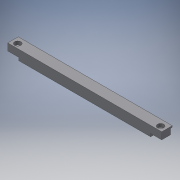
# Autodesk Inventor part: Case_bottom_front
Saved by Autodesk Inventor 2016 SP2 (Build 200236200, 236)
## iProperties
Created: 2018-06-26
Part Number: Case_bottom_front
Material: Generisch
Document SubType Name: Modeling
Designer: Nils
Density: 1 g/cm^3
Appearance: Vorgabe
Author: Nils
Autodesk Inventor part; units mm, degrees
ref_plane "YZ Plane" through (0, 0, 0) normal (1, 0, 0) x (0, 1, 0)
ref_plane "XZ Plane" through (0, 0, 0) normal (0, 1, 0) x (-1, 0, 0)
ref_plane "XY Plane" through (0, 0, 0) normal (0, 0, 1) x (1, 0, 0)
sketch "Skizze2" plane through (0, 0, 0) normal (1, 0, 0) x (0, 1, 0)
  line L0 (-333.777, 348.0872) -> (-334.0423, 350.6737)
  line L1 (-333.777, 348.0872) -> (-333.134, 341.8201)
  line L2 (-333.134, 341.8201) -> (-342.5844, 340.8506)
  line L3 (-342.0005, 349.8573) -> (-334.0423, 350.6737)
  line L4 (-342.7069, 342.0444) -> (-341.2147, 342.1975)
  line L5 (-342.7069, 342.0444) -> (-342.5844, 340.8506)
  line L6 (-333.134, 341.8201) -> (-342.5844, 340.8506)
  line L7 (-333.777, 348.0872) -> (-333.134, 341.8201)
  line L8 (-333.777, 348.0872) -> (-341.7352, 347.2708)
  line L9 (-341.2147, 342.1975) -> (-341.7352, 347.2708)
  line L10 (-342.7069, 342.0444) -> (-342.5844, 340.8506)
  line L11 (-341.7352, 347.2708) -> (-342.0005, 349.8573)
  point P0 (0, 0)
extrude "Extrusion1" add sketch "Skizze2" along normal blind 69.4
sketch "Skizze3" plane through (0, 0, 0) normal (-1, 0, 0) x (0, 0, 1)
  line L0 (342.0444, -342.7069) -> (342.1975, -341.2147) projected
  line L1 (342.0444, -342.7069) -> (340.8506, -342.5844) projected
  line L2 (341.8201, -333.134) -> (340.8506, -342.5844) projected
  line L3 (348.0872, -333.777) -> (341.8201, -333.134) projected
  line L4 (348.0872, -333.777) -> (347.2708, -341.7352) projected
  line L5 (342.1975, -341.2147) -> (347.2708, -341.7352) projected
  line L6 (350.6737, -334.0423) -> (349.8573, -342.0005) projected
  line L7 (349.8573, -342.0005) -> (348.0872, -342.0005)
  line L8 (348.0872, -342.0005) -> (348.0872, -333.777)
  line L9 (348.0872, -333.777) -> (349.8573, -333.777)
  line L10 (349.8573, -333.777) -> (349.8573, -342.0005)
  point P0 (0, 0)
  constraints: 8 end point, 2 parallel, 1 horizontal, 1 perpendicular
extrude "Extrusion2" cut sketch "Skizze3" against normal blind 10 contours L9 L10 L7 L8
sketch "Skizze4" plane through (0, -333.134, 341.8201) normal (0, 0.1020498, -0.9947793) x (1, 0, 0)
  line L0 (0, 0) -> (10, 0) construction
  line L1 (5, 0) -> (5, 9.5) construction
  line L2 (0, 9.5) -> (69.4, 9.5) construction
  circle A0 centre (5, 4) radius 2.85
  line L3 (0, 9.5) -> (0, 0) construction
  point P0 (0, -296.5122)
  point P1 (0, 8.4553)
  point P2 (0, 8.913)
  dimension "d4" = 5.7
  dimension "d5" = 5
  dimension "d6" = 4
  constraints: 2 end point, 2 point on line, 1 centre point, 1 midpoint, 1 vertical
  measures "d4" diameter of A0
  measures "d5" distance between parallel lines of L3 L1
  measures "d6" distance from line of L0 A0.centre
extrude "Extrusion3" cut sketch "Skizze4" against normal blind 3.1
sketch "Skizze5" plane through (5, -337.4295, 344.4957) normal (0, 0.1020498, -0.9947793) x (-1, 0, 0)
  circle A0 centre (0, 0) radius 2.85 projected
  circle A1 centre (0, 0) radius 1.5
  point P0 (5, 300.5122)
  dimension "d9" = 3
  constraints: 1 centre point, 1 coincident
  measures "d9" diameter of A1
extrude "Extrusion4" cut sketch "Skizze5" against normal blind 3.4 contours A1
mirror "Spiegeln1" about plane through (69.4, -337.8887, 348.9722) normal (1, 0, 0) of "Extrusion4", "Extrusion3", "Extrusion2", "Extrusion1"
